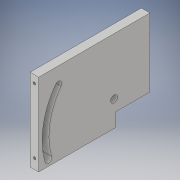
# Autodesk Inventor part: third odomitry wheel
Saved by Autodesk Inventor 2019 (Build 230136000, 136)
## iProperties
Created: 2020-10-13
Part Number: third odomitry wheel
Material: Generic
Document SubType Name: Modeling
Designer: User
Density: 1 g/cm^3
Appearance: Default
Author: User
Autodesk Inventor part; units mm, degrees
ref_plane "YZ Plane" through (0, 0, 0) normal (1, 0, 0) x (0, 1, 0)
ref_plane "XZ Plane" through (0, 0, 0) normal (0, 1, 0) x (-1, 0, 0)
ref_plane "XY Plane" through (0, 0, 0) normal (0, 0, 1) x (1, 0, 0)
sketch "Sketch1" plane through (0, 0, 0) normal (1, 0, 0) x (0, 1, 0)
  line L0 (0, 0) -> (50.8, 0)
  line L1 (50.8, 0) -> (50.8, -82.55)
  line L2 (50.8, -82.55) -> (0, -82.55)
  line L3 (0, -82.55) -> (0, -57.15)
  line L4 (0, -57.15) -> (-10.16, -57.15)
  line L5 (-10.16, -57.15) -> (-10.16, 0)
  line L6 (-10.16, 0) -> (0, 0)
  dimension "d0" = 82.55
  dimension "d1" = 50.8
  dimension "d27" = 25.4
  dimension "d28" = 10.16
  constraints: 14 end point, 4 perpendicular, 1 horizontal, 1 parallel, 1 vertical
  measures "d0" distance of L0.end L1.end
  measures "d1" distance of L1.end L2.end
  measures "d27" distance of L2.end L3.end
  measures "d28" distance of L3.end L4.end
extrude "Extrusion1" add sketch "Sketch1" along normal blind 6.35
sketch "Sketch2" plane through (6.35, 0, 0) normal (1, 0, 0) x (0, 0, -1)
  circle A0 centre (55.88, 8.89) radius 2.54
  line L0 (0, 0) -> (25.4, 0) projected
  line L1 (0, 50.8) -> (0, 0) projected
  line L2 (57.15, -10.16) -> (57.15, 0) projected
  arc A1 (14.5266, 38.3949) -> (7.2244, -5.7138) centre (55.88, 8.89) ccw construction
  arc A2 (12.459, 39.8702) -> (4.7916, -6.444) centre (55.88, 8.89) ccw
  arc A3 (16.5943, 36.9197) -> (9.6572, -4.9836) centre (55.88, 8.89) ccw
  arc A4 (16.5943, 36.9197) -> (12.459, 39.8702) centre (14.5266, 38.3949) ccw
  arc A5 (4.7916, -6.444) -> (9.6572, -4.9836) centre (7.2244, -5.7138) ccw
  point P0 (82.55, 0)
  dimension "d4" = 8.89
  dimension "d7" = 5.08
  dimension "d43" = 1.27
  dimension "d44" = 52.214
  dimension "d46" = 2.54
  dimension "d47" = 50.8
  constraints: 10 point on circle, 6 centre point, 4 tangent, 1 coincident
  measures "d4" distance from line of L0 A0.centre
  measures "d7" diameter of A0
  measures "d43" distance from line of A0.centre L2
  measures "d46" radius of A4
  measures "d47" radius of A1
extrude "Extrusion2" cut sketch "Sketch2" against normal through all
sketch "Sketch6" plane through (0, 0, -82.55) normal (0, -1, 0) x (1, 0, 0)
  line L0 (0, 0) -> (0, 25.4) projected
  line L1 (0, 0) -> (0, 25.4) projected
  line L2 (0, 0) -> (6.35, 0) projected
  line L3 (6.35, 25.4) -> (6.35, 0) projected
  line L4 (0, 25.4) -> (6.35, 25.4) projected
  point P0 (0, 82.55)
  point P1 (3.175, 12.7)
sketch "Sketch7" plane through (0, -10.16, 0) normal (0, 0, 1) x (1, 0, 0)
  line L0 (0, 0) -> (0, 60.96) projected
  line L1 (0, 0) -> (6.35, 0) projected
  line L2 (6.35, 60.96) -> (6.35, 0) projected
  line L3 (0, 60.96) -> (6.35, 60.96) projected
  point P0 (0, 10.16)
  point P1 (3.3657, 7.358)
  point P2 (3.175, 55.3802)
hole "Hole2" at (3.175, 0, -69.85) direction (0, 1, 0) diameter 1.9304 depth 7.6708 tip angle 118
hole "Hole3" at (3.3657, -2.802, 0) at (3.175, 45.2202, 0) direction (0, 0, -1) diameter 1.9304 depth 7.6708 tip angle 118
body "Solid1"
